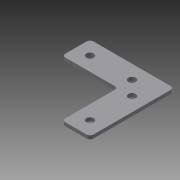
# Autodesk Inventor part: Gusset Connector
Saved by Autodesk Inventor 2013 (Build 170138000, 138)
## iProperties
Created: 2013-01-26
Part Number: Gusset Connector
Material: Generic
Document SubType Name: Modeling
Designer: actoennies
Density: 1 g/cm^3
Author: actoennies
Autodesk Inventor part; units mm, degrees
ref_plane "YZ Plane" through (0, 0, 0) normal (1, 0, 0) x (0, 1, 0)
ref_plane "XZ Plane" through (0, 0, 0) normal (0, 1, 0) x (-1, 0, 0)
ref_plane "XY Plane" through (0, 0, 0) normal (0, 0, 1) x (1, 0, 0)
sketch "Sketch1" plane through (0, 0, 0) normal (0, 1, 0) x (-1, 0, 0)
  line L0 (0, 3.175) -> (0, 73.025)
  line L1 (3.175, 76.2) -> (22.225, 76.2)
  line L2 (25.4, 73.025) -> (25.4, 28.575)
  line L3 (28.575, 25.4) -> (73.025, 25.4)
  line L4 (76.2, 22.225) -> (76.2, 3.175)
  line L5 (73.025, 0) -> (3.175, 0)
  line L6 (25.4, 25.4) -> (0, 0) construction
  circle A0 centre (12.7, 63.5) radius 3.3782
  circle A1 centre (12.7, 25.4) radius 3.3782
  circle A2 centre (25.4, 12.7) radius 3.3782
  circle A3 centre (63.5, 12.7) radius 3.3782
  arc A4 (3.175, 76.2) -> (0, 73.025) centre (3.175, 73.025) ccw
  arc A5 (25.4, 73.025) -> (22.225, 76.2) centre (22.225, 73.025) ccw
  arc A6 (0, 3.175) -> (3.175, 0) centre (3.175, 3.175) ccw
  arc A7 (25.4, 28.575) -> (28.575, 25.4) centre (28.575, 28.575) ccw
  arc A8 (76.2, 22.225) -> (73.025, 25.4) centre (73.025, 22.225) ccw
  arc A9 (73.025, 0) -> (76.2, 3.175) centre (73.025, 3.175) ccw
  point P0 (0, 76.2)
  point P1 (25.4, 76.2)
  point P2 (76.2, 25.4)
  point P3 (76.2, 0)
  dimension "d0" = 76.2
  dimension "d1" = 25.4
  dimension "d2" = 50.8
  dimension "d3" = 50.8
  dimension "d4" = 25.4
  dimension "d5" = 6.7564
  dimension "d6" = 6.7564
  dimension "d7" = 6.7564
  dimension "d8" = 6.7564
  dimension "d9" = 12.7
  dimension "d10" = 0
  dimension "d11" = 12.7
  dimension "d12" = 12.7
  dimension "d13" = 12.7
  dimension "d14" = 12.7
  dimension "d15" = 12.7
  dimension "d16" = 3.175
  constraints: 14 end point, 13 point on line, 12 point on circle, 12 tangent, 10 centre point, 5 equal radius, 3 parallel, 1 perpendicular, 1 vertical
  measures "d0" distance of L6.end point (0, 76.2)
  measures "d1" distance of point (0, 76.2) point (25.4, 76.2)
  measures "d2" distance of point (25.4, 76.2) L6.start
  measures "d3" distance of L6.start point (76.2, 25.4)
  measures "d4" distance of point (76.2, 25.4) point (76.2, 0)
  measures "d5" diameter of A0
  measures "d6" diameter of A1
  measures "d7" diameter of A2
  measures "d8" diameter of A3
  measures "d9" distance from line of L5 A2.centre
  measures "d10" distance from line of L3 A1.centre
  measures "d11" distance from line of L2 A1.centre
  measures "d12" distance from line of L4 A3.centre
  measures "d13" distance from line of L5 A3.centre
  measures "d14" distance from line of L1 A0.centre
  measures "d15" distance from line of L2 A0.centre
  measures "d16" radius of A4
extrude "Extrusion1" add sketch "Sketch1" along normal blind 3.175
body "Solid1"
